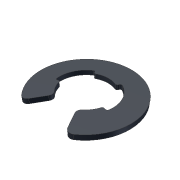
# Autodesk Inventor part: anel_elastico
Saved by Autodesk Inventor 2012 SP2 (Build 160219200, 219)
## iProperties
Created: 2015-04-29
Part Number: anel_elastico
Material: Padrão
Document SubType Name: Chapa
Designer: Projeto02
Density: 1 g/cm^3
Sheet Metal Rule: Padrão_mm
Author: Projeto02
Autodesk Inventor part; units mm, degrees
ref_plane "YZ Plane" through (0, 0, 0) normal (1, 0, 0) x (0, 1, 0)
ref_plane "XZ Plane" through (0, 0, 0) normal (0, 1, 0) x (-1, 0, 0)
ref_plane "XY Plane" through (0, 0, 0) normal (0, 0, 1) x (1, 0, 0)
sketch "Esboço1" plane through (0, 0, 0) normal (0, 0, 1) x (1, 0, 0)
  arc A0 (5, -8.6603) -> (-5, -8.6603) centre (0, 0) ccw
  line L0 (0, 0) -> (3, 0)
  line L1 (0, 0) -> (3, 0) construction
  line L2 (-2.5, -4.3301) -> (-5, -8.6603)
  line L3 (2.5, -4.3301) -> (5, -8.6603)
  line L4 (-2.5, 4.3301) -> (-3, 5.1962)
  line L5 (2.5, 4.3301) -> (3, 5.1962)
  arc A1 (-3, 5.1962) -> (-5.7956, -1.5529) centre (0, 0) ccw
  arc A2 (5.7956, -1.5529) -> (3, 5.1962) centre (0, 0) ccw
  arc A3 (-4.8296, -1.2941) -> (-2.5, -4.3301) centre (0, 0) ccw
  arc A4 (2.5, -4.3301) -> (4.8296, -1.2941) centre (0, 0) ccw
  arc A5 (2.5, 4.3301) -> (-2.5, 4.3301) centre (0, 0) ccw
  line L6 (-4.8296, -1.2941) -> (-5.7956, -1.5529)
  line L7 (4.8296, -1.2941) -> (5.7956, -1.5529)
  dimension "d3" = 3
  dimension "d4" = 0
  dimension "d5" = 60
  dimension "d6" = 60
  dimension "d9" = 45
  dimension "d10" = 45
  dimension "d11" = 5
  dimension "d12" = 5
  dimension "d13" = 6
  dimension "d14" = 6
  dimension "d15" = 5
  dimension "d20" = 4
  measures "d3" distance of L0.start L0.end
  measures "d4" distance between parallel lines of L0 L1
  measures "d5" angle of L3 L2
  measures "d6" angle of L0 L3
  measures "d9" angle of L2 L6
  measures "d10" angle of L7 L3
  measures "d11" radius of A4
  measures "d12" radius of A5
  measures "d13" radius of A1
  measures "d14" radius of A2
  measures "d15" radius of A3
  measures "d20" radial gap between concentric circles of A1 A0
extrude "Placa1" add sketch "Esboço1" along normal blind 1
fillet "Arredondamento de canto1" radius 1 4 edges at (-2.5, -4.3301, 0.5) (-5, -8.6603, 0.5) (5, -8.6603, 0.5) (2.5, -4.3301, 0.5)
fillet "Arredondamento de canto2" radius 0.35 8 edges at (-4.8296, -1.2941, 0.5) (-5.7956, -1.5529, 0.5) (-2.5, 4.3301, 0.5) (-3, 5.1962, 0.5) (2.5, 4.3301, 0.5) (3, 5.1962, 0.5) (5.7956, -1.5529, 0.5) (4.8296, -1.2941, 0.5)
equation "\"d12\" = d15"
equation "\"d13\" = d14"
equation "\"d15\" = d11"
equation "\"Raio_dobra\" = Espessura"
equation "\"Largura_alívio_de_dobra\" = Espessura"
equation "\"Profundidade_alívio_de_dobra\" = 0.5 * Espessura"
equation "\"Tamanho_alívio_de_dobra\" = 4 * Espessura"
equation "\"Remanescente_mínimo\" = 2 * Espessura"
equation "\"Raiodetransição\" = Raio_dobra"
equation "\"Tamanho_de_raio_de_Jacobi\" = Raio_dobra"
equation "\"TamanhoFolga\" = Espessura"
equation "\"d8\" = d7"
equation "\"d17\" = Raio_dobra"
equation "\"Espessura\" = 1"
equation "\"d7\" = 45deg"
